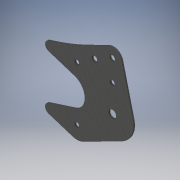
# Autodesk Inventor part: Shooter Side Plate
Saved by Autodesk Inventor 2019.4 (Build 234330000, 330)
## iProperties
Created: 2020-01-16
Part Number: Shooter Side Plate
Material: CFRP
Document SubType Name: Modeling
Designer: admin
Density: 1.43 g/cm^3
Appearance: Carbon Fiber
Mass: 627.814 g
Surface Area: 1851.62 cm^2
Volume: 439.031 cm^3
Author: admin
Autodesk Inventor part; units mm, degrees
ref_plane "YZ Plane" through (0, 0, 0) normal (1, 0, 0) x (0, 1, 0)
ref_plane "XZ Plane" through (0, 0, 0) normal (0, 1, 0) x (-1, 0, 0)
ref_plane "XY Plane" through (0, 0, 0) normal (0, 0, 1) x (1, 0, 0)
sketch "Sketch1" plane through (0, 0, 0) normal (0, 0, 1) x (1, 0, 0)
  circle A0 centre (-150, -114.3) radius 50.8 construction
  circle A1 centre (-150, 114.3) radius 50.8 construction
  line L0 (-150, 114.3) -> (-150, -114.3) construction
  line L1 (-150, 0) -> (0, 0) construction
  circle A2 centre (0, 114.3) radius 50.8 construction
  line L2 (0, 0) -> (0, 114.3) construction
  circle A3 centre (0, 0) radius 88.9 construction
  circle A4 centre (-75, 164.0494) radius 32.5 construction
  circle A5 centre (-75, 164.0494) radius 11
  line L3 (0, 0) -> (-368.1737, 0) construction
  circle A6 centre (-0.1342, 204.2999) radius 32.5 construction
  circle A7 centre (-0.1342, 204.2999) radius 11
  line L4 (-75, 164.0494) -> (0, 114.3) construction
  line L5 (-75, 164.0494) -> (-150, 114.3) construction
  line L6 (-0.1342, 204.2999) -> (-75, 164.0494) construction
  line L7 (-0.1342, 204.2999) -> (0, 114.3) construction
  circle A8 centre (0, 114.3) radius 9.5
  circle A9 centre (0, 0) radius 16
  circle A10 centre (-150, -114.3) radius 9.5
  circle A11 centre (-150, -114.3) radius 25 construction
  circle A12 centre (-150, 114.3) radius 9.5
  arc A13 (-163.9628, 61.1019) -> (-174.1656, 163.7067) centre (-150, 114.3) ccw construction
  arc A14 (-17.7091, 240.2321) -> (38.6968, 213.8996) centre (-0.1342, 204.2999) ccw construction
  line L8 (-174.1656, 163.7067) -> (-17.7091, 240.2321)
  line L9 (-330, 114.3) -> (-166.8056, 61.9304)
  arc A15 (-125.0719, -163.3264) -> (-163.9628, -61.1019) centre (-150, -114.3) ccw construction
  line L10 (-166.8056, -61.9304) -> (-330, -114.3)
  line L11 (-330, -114.3) -> (-166.8056, -166.6696)
  line L12 (38.6968, 213.8996) -> (103.2528, -47.2317)
  line L13 (103.2528, -47.2317) -> (-125.0719, -163.3264)
  line L14 (-330, -114.3) -> (-150, -114.3) construction
  line L15 (-330, 114.3) -> (-150, 114.3) construction
  line L16 (-330, 114.3) -> (-174.1656, 163.7067)
  arc A16 (-163.9628, -61.1019) -> (-163.9628, 61.1019) centre (-180, 0) ccw
  arc A17 (38.6968, 213.8996) -> (-17.7091, 240.2321) centre (-0.1342, 204.2999) ccw
  arc A18 (-166.8056, -166.6696) -> (-125.0719, -163.3264) centre (-150, -114.3) ccw
  arc A19 (-166.8056, -61.9304) -> (-166.8056, -166.6696) centre (-150, -114.3) ccw construction
  arc A20 (-163.9628, -61.1019) -> (-166.8056, -61.9304) centre (-150, -114.3) ccw
  arc A21 (-166.8056, 61.9304) -> (-163.9628, 61.1019) centre (-150, 114.3) ccw
  arc A22 (-174.1656, 163.7067) -> (-166.8056, 61.9304) centre (-150, 114.3) ccw construction
  dimension "d0" = 101.6
  dimension "d1" = 101.6
  dimension "d3" = 101.6
  dimension "d4" = 228.6
  dimension "d5" = 114.3
  dimension "d6" = 177.8
  dimension "d7" = 150
  dimension "d9" = 65
  dimension "d11" = 22
  dimension "d13" = 0
  dimension "d14" = 65
  dimension "d15" = 22
  dimension "d16" = 90
  dimension "d17" = 90
  dimension "d18" = 85
  dimension "d19" = 90
  dimension "d20" = 19
  dimension "d21" = 32
  dimension "d22" = 19
  dimension "d23" = 50
  dimension "d24" = 19
  dimension "d25" = 110
  dimension "d26" = 80
  dimension "d27" = 110
  dimension "d28" = 180
  dimension "d29" = 180
  dimension "d30" = 30
  constraints: 34 end point, 23 centre point, 21 point on circle, 18 tangent, 10 coincident, 3 horizontal, 2 perpendicular, 1 midpoint
  measures "d0" diameter of A0
  measures "d1" diameter of A1
  measures "d3" diameter of A2
  measures "d4" distance of L0.start L0.end
  measures "d5" distance of L1.end L2.end
  measures "d6" diameter of A3
  measures "d7" distance of L1.start L1.end
  measures "d9" diameter of A4
  measures "d11" diameter of A5
  measures "d13" distance between parallel lines of L3 L1
  measures "d14" diameter of A6
  measures "d15" diameter of A7
  measures "d16" distance of L4.start L2.end
  measures "d17" distance of L4.start L0.start
  measures "d18" distance of L6.start L4.start
  measures "d19" distance of L6.start L2.end
  measures "d20" diameter of A8
  measures "d21" diameter of A9
  measures "d22" diameter of A10
  measures "d23" diameter of A11
  measures "d24" diameter of A12
  measures "d25" diameter of A13
  measures "d26" diameter of A14
  measures "d27" diameter of A15
  measures "d28" distance of A12.centre L9.start
  measures "d29" distance of A10.centre L10.end
  measures "d30" distance of L1.start A16.centre
extrude "Extrusion1" add sketch "Sketch1" along normal blind 5
fillet "Fillet1" radius 20 2 edges at (-330, 114.3, 2.5) (-330, -114.3, 2.5)
fillet "Fillet2" radius 88.9 1 edges at (103.2528, -47.2317, 2.5)
fillet "Fillet3" radius 1000 1 edges at (-174.1656, 163.7067, 2.5)
body "Solid1"
